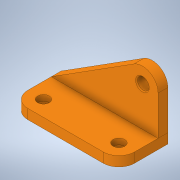
# Autodesk Inventor part: Pieza13
Saved by Autodesk Inventor 2020 (Build 240168000, 168)
## iProperties
Created: 2020-02-28
Part Number: Pieza13
Material: Cobre
Document SubType Name: Modeling
Designer: Linda
Density: 8.94 g/cm^3
Appearance: Naranja
Author: Linda
Autodesk Inventor part; units mm, degrees
ref_plane "YZ Plane" through (0, 0, 0) normal (1, 0, 0) x (0, 1, 0)
ref_plane "XZ Plane" through (0, 0, 0) normal (0, 1, 0) x (-1, 0, 0)
ref_plane "XY Plane" through (0, 0, 0) normal (0, 0, 1) x (1, 0, 0)
sketch "Boceto1" plane through (0, 0, 0) normal (0, 0, 1) x (1, 0, 0)
  circle A0 centre (46.519, 19.9996) radius 3
  arc A1 (54.519, 20) -> (42.2378, 26.7576) centre (46.519, 19.9996) ccw
  line L0 (54.52, 0) -> (54.519, 20)
  line L1 (0, 0) -> (42.2378, 26.7576)
  line L2 (0, 0) -> (0, -5)
  line L3 (0, -5) -> (54.52, -5)
  line L4 (54.52, -5) -> (54.52, 0)
  dimension "d5" = 50
  dimension "d6" = 20
  dimension "d8" = 5
  dimension "d9" = 54.52
  constraints: 10 end point, 2 centre point, 2 perpendicular, 2 point on circle, 2 tangent, 1 coincident, 1 vertical
  measures "d5" distance of L1.start L1.end
  measures "d6" distance of L0.start L0.end
  measures "d8" distance of L1.start L2.end
  measures "d9" distance of L2.end L3.end
extrude "Extrusión1" add sketch "Boceto1" along normal blind 5
sketch "Boceto2" plane through (0, 0, 5) normal (0, 0, 1) x (1, 0, 0)
  line L0 (0, 0) -> (0, -5) projected
  line L1 (0, 0) -> (0, -5)
  line L2 (0, -5) -> (54.52, -5) projected
  line L3 (0, -5) -> (54.52, -5)
  line L4 (54.52, -5) -> (54.52, 0) projected
  line L5 (54.52, -5) -> (54.52, 0)
  line L6 (54.52, 0) -> (0, 0)
  constraints: 8 end point, 3 perpendicular, 1 vertical
extrude "Extrusión2" add sketch "Boceto2" along normal blind 20
fillet "Empalme1" radius 8 2 edges at (54.52, -2.5, 25) (0, -2.5, 25)
sketch "Boceto3" plane through (0, 0, 5) normal (0, 1, 0) x (1, 0, 0)
  circle A0 centre (8, -12) radius 3
  circle A1 centre (46.52, -12) radius 3
  point P0 (0, 5)
  dimension "d15" = 6
  dimension "d16" = 6
  constraints: 2 centre point
  measures "d15" diameter of A0
  measures "d16" diameter of A1
hole "Agujero1" at (8, 0, 17) at (46.52, 0, 17) direction (0, -1, 0) diameter 6 depth 3 tip angle 118
sketch "Boceto4" plane through (0, 0, 5) normal (0, 1, 0) x (1, 0, 0)
  circle A0 centre (8, -12) radius 3 projected
  circle A1 centre (46.52, -12) radius 3 projected
  point P0 (0, 5)
hole "Agujero2" at (46.52, 0, 17) at (8, 0, 17) direction (0, -1, 0) diameter 4 depth 5 tip angle 118
chamfer "Chaflán1" distance 0.5 angle 45 1 edges at (43.519, 19.9996, 5) measured on face at (43.019, 19.9996, 5)
